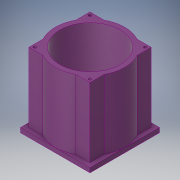
# Autodesk Inventor part: 000.201 - Станина
Saved by Autodesk Inventor 2019 (Build 230136000, 136)
## iProperties
Created: 2020-03-17
Part Number: 000.201 - Станина
Material: Пластик АБС
Document SubType Name: Modeling
Designer: Петров Иван
Density: 1.06 g/cm^3
Appearance: Гладкий — пурпурный
Author: Петров Иван
Autodesk Inventor part; units mm, degrees
ref_plane "YZ Plane" through (0, 0, 0) normal (1, 0, 0) x (0, 1, 0)
ref_plane "XZ Plane" through (0, 0, 0) normal (0, 1, 0) x (-1, 0, 0)
ref_plane "XY Plane" through (0, 0, 0) normal (0, 0, 1) x (1, 0, 0)
sketch "Эскиз1" plane through (0, 0, 0) normal (0, 1, 0) x (-1, 0, 0)
  line L0 (-75, 75) -> (75, 75)
  line L1 (75, 75) -> (75, -75)
  line L2 (75, -75) -> (-75, -75)
  line L3 (-75, -75) -> (-75, 75)
  line L4 (-75, 75) -> (75, -75) construction
  line L5 (75, 75) -> (-75, -75) construction
  point P0 (0, 0)
  dimension "d0" = 150
  dimension "d1" = 150
  constraints: 12 end point, 2 midpoint, 2 parallel, 1 horizontal, 1 perpendicular
  measures "d0" distance of L1.end L2.end
  measures "d1" distance of L0.end L1.end
extrude "Выдавливание1" add sketch "Эскиз1" along normal blind 10
sketch "Эскиз2" plane through (0, 10, 0) normal (0, 1, 0) x (1, 0, 0)
  circle A0 centre (0, 0) radius 75
  circle A1 centre (0, 0) radius 65
  dimension "d4" = 150
  dimension "d5" = 130
  constraints: 2 centre point, 2 coincident
  measures "d4" diameter of A0
  measures "d5" diameter of A1
extrude "Выдавливание2" add sketch "Эскиз2" along normal blind 150
sketch "Эскиз3" plane through (0, 10, 0) normal (0, 1, 0) x (1, 0, 0)
  line L0 (0, 0) -> (-53.033, -53.033)
  arc A0 (-75, 0) -> (0, -75) centre (0, 0) ccw projected
  line L1 (0, 0) -> (75, 0) construction
  line L2 (-53.033, -53.033) -> (-66.033, -53.033)
  line L3 (-66.033, -53.033) -> (-66.033, -66.033)
  line L4 (-66.033, -66.033) -> (-53.033, -66.033)
  line L5 (-53.033, -66.033) -> (-53.033, -53.033)
  line L6 (-53.033, -66.033) -> (-35.5618, -66.033)
  line L7 (-66.033, -53.033) -> (-66.033, -35.5618)
  arc A1 (-66.033, -35.5618) -> (-35.5618, -66.033) centre (0, 0) ccw
  circle A2 centre (-59.533, -59.533) radius 3
  dimension "d8" = 135
  dimension "d9" = 13
  dimension "d10" = 13
  dimension "d11" = 6
  dimension "d12" = 6.5
  dimension "d13" = 6.5
  constraints: 16 end point, 6 point on circle, 3 horizontal, 2 centre point, 2 parallel, 2 perpendicular, 1 equal length
  measures "d8" angle of L0 L1
  measures "d9" distance of L4.end L3.end
  measures "d10" distance of L3.end L2.end
  measures "d11" diameter of A2
  measures "d12" distance from line of L3 A2.centre
  measures "d13" distance from line of L4 A2.centre
extrude "Выдавливание3" add sketch "Эскиз3" along normal up to surface (150 mm away)
pattern_circular "Круговой массив1" count 4 over 360 about axis through (0, 10, 0) along (0, 1, 0) of "Выдавливание3"
